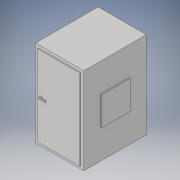
# Autodesk Inventor part: enclosureNode
Saved by Autodesk Inventor 2017 (Build 210142000, 142)
## iProperties
Created: 2016-06-20
Part Number: enclosureNode
Material: Generic
Document SubType Name: Modeling
Designer: Zuhra Abdurashidova
Density: 1 g/cm^3
Appearance: Default
Author: Zuhra Abdurashidova
Autodesk Inventor part; units mm, degrees
ref_plane "YZ Plane" through (0, 0, 0) normal (1, 0, 0) x (0, 1, 0)
ref_plane "XZ Plane" through (0, 0, 0) normal (0, 1, 0) x (-1, 0, 0)
ref_plane "XY Plane" through (0, 0, 0) normal (0, 0, 1) x (1, 0, 0)
sketch "Sketch1" plane through (0, 0, 0) normal (0, 1, 0) x (-1, 0, 0)
  point P0 (0, 0)
sketch "Sketch2" plane through (0, 0, 0) normal (0, 1, 0) x (-1, 0, 0)
  line L0 (-250, 325) -> (250, 325)
  line L1 (250, 325) -> (250, -325)
  line L2 (250, -325) -> (-250, -325)
  line L3 (-250, -325) -> (-250, 325)
  line L4 (-250, 325) -> (250, -325) construction
  line L5 (250, 325) -> (-250, -325) construction
  point P0 (0, 0)
  dimension "d16" = 650
  dimension "d17" = 500
  constraints: 12 end point, 2 midpoint, 2 parallel, 1 horizontal, 1 perpendicular
  measures "d16" distance of L0.end L1.end
  measures "d17" distance of L1.end L2.end
extrude "Node" add sketch "Sketch2" along normal blind 900
shell "Shell1" thickness 30 removed faces 0
sketch "Sketch3" plane through (-250, 0, 325) normal (0, 0, 1) x (1, 0, 0)
  line L0 (30, 30) -> (470, 30)
  line L1 (470, 30) -> (470, 870)
  line L2 (470, 870) -> (30, 870)
  line L3 (30, 870) -> (30, 30)
  line L4 (30, 30) -> (470, 870) construction
  line L5 (470, 30) -> (30, 870) construction
  line L6 (500, 0) -> (500, 900) projected
  line L7 (0, 900) -> (500, 900) projected
  line L8 (0, 0) -> (0, 900) projected
  line L9 (500, 0) -> (0, 0) projected
  point P0 (250, 0)
  point P1 (250, 450)
  dimension "d21" = 30
  dimension "d22" = 30
  dimension "d23" = 30
  dimension "d24" = 30
  constraints: 12 end point, 2 midpoint, 2 parallel, 1 horizontal, 1 perpendicular
  measures "d21" distance between parallel lines of L6 L1
  measures "d22" distance between parallel lines of L7 L2
  measures "d23" distance between parallel lines of L8 L3
  measures "d24" distance between parallel lines of L9 L0
extrude "Door" add sketch "Sketch3" along normal blind 10 contours L3 L2 L1 L0
sketch "Sketch4" plane through (250, 0, 325) normal (1, 0, 0) x (0, 0, -1)
  line L0 (176.8638, 304.0117) -> (476.8638, 304.0117)
  line L1 (476.8638, 304.0117) -> (476.8638, 604.0117)
  line L2 (476.8638, 604.0117) -> (176.8638, 604.0117)
  line L3 (176.8638, 604.0117) -> (176.8638, 304.0117)
  line L4 (176.8638, 304.0117) -> (476.8638, 604.0117) construction
  line L5 (476.8638, 304.0117) -> (176.8638, 604.0117) construction
  point P0 (325, 0)
  point P1 (326.8638, 454.0117)
  dimension "d27" = 300
  dimension "d28" = 300
  constraints: 12 end point, 2 midpoint, 2 parallel, 1 horizontal, 1 perpendicular
  measures "d27" distance of L1.end L2.end
  measures "d28" distance of L0.end L1.end
extrude "SMA pannel" add sketch "Sketch4" along normal blind 10
sketch "Sketch5" plane through (-250, 0, 335) normal (0, 0, 1) x (1, 0, 0)
  line L0 (59.5914, 457.1317) -> (79.5601, 457.1317)
  line L1 (79.5601, 457.1317) -> (79.5601, 442.8683)
  line L2 (79.5601, 442.8683) -> (59.5914, 442.8683)
  line L3 (59.5914, 442.8683) -> (59.5914, 457.1317)
  line L4 (59.5914, 457.1317) -> (79.5601, 442.8683) construction
  line L5 (79.5601, 457.1317) -> (59.5914, 442.8683) construction
  point P0 (250, 0)
  point P1 (69.5757, 450)
  constraints: 12 end point, 2 midpoint, 2 parallel, 1 horizontal, 1 perpendicular
extrude "handle1" add sketch "Sketch5" along normal blind 20
sketch "Sketch6" plane through (-170.4399, 442.8683, 335) normal (1, 0, 0) x (0, 0, -1)
  line L0 (-20, 14.2634) -> (-12.9022, 14.2634)
  line L1 (-12.9022, 14.2634) -> (-12.9022, -0.0578)
  line L2 (-12.9022, -0.0578) -> (-20, -0.0578)
  line L3 (-20, -0.0578) -> (-20, 14.2634)
  point P0 (335, -442.8683)
  constraints: 8 end point, 2 parallel, 1 horizontal, 1 perpendicular
extrude "handle2" add sketch "Sketch6" along normal blind 50
body "Solid2"
